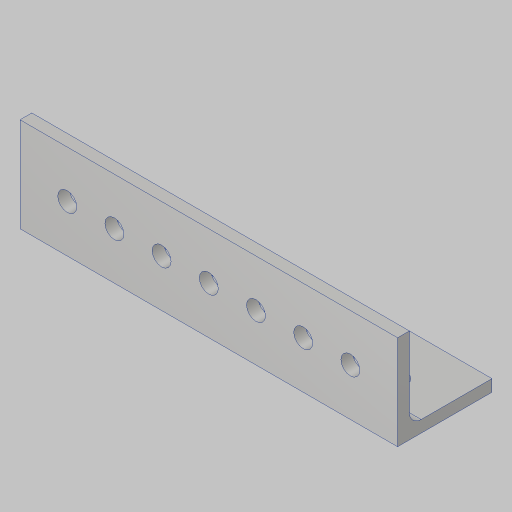
# Autodesk Inventor part: GI - 008
Saved by Autodesk Inventor 2023.5 (Build 275446000, 446)
## iProperties
Created: 2025-01-26
Part Number: GI - 008
Material: Aluminum 6061
Document SubType Name: Modeling
Designer: slick
Density: 2.7 g/cm^3
Appearance: Aluminum - Flat
Author: slick
Autodesk Inventor part; units mm, degrees
ref_plane "YZ Plane" through (0, 0, 0) normal (1, 0, 0) x (0, 1, 0)
ref_plane "XZ Plane" through (0, 0, 0) normal (0, 1, 0) x (-1, 0, 0)
ref_plane "XY Plane" through (0, 0, 0) normal (0, 0, 1) x (1, 0, 0)
sketch "Sketch1" plane through (0, 0, 0) normal (1, 0, 0) x (0, 1, 0)
  line L0 (25.4, 0) -> (0, 0)
  line L1 (0, 0) -> (0, -25.4)
  line L2 (0, -25.4) -> (3.175, -25.4)
  line L3 (3.175, -25.4) -> (3.175, -3.175)
  line L4 (3.175, -3.175) -> (25.4, -3.175)
  line L5 (25.4, -3.175) -> (25.4, 0)
  dimension "d0" = 25.4
  dimension "d1" = 25.4
  dimension "d2" = 3.175
  constraints: 12 end point, 5 perpendicular, 1 horizontal, 1 vertical
  measures "d0" distance of L0.start L0.end
  measures "d1" distance of L0.end L1.end
  measures "d2" distance between parallel lines of L4 L0
extrude "Extrusion1" add sketch "Sketch1" along normal mid plane 101.6
fillet "Fillet1" radius 3.175 1 edges at (0, 3.175, -3.175)
sketch "Sketch2" plane through (-50.8, 0, 0) normal (0, 0, 1) x (1, 0, 0)
  line L0 (0, 0) -> (0, 25.4) projected
  line L1 (101.6, 0) -> (0, 0) projected
  point P0 (50.8, 0)
  point P1 (12.7, 12.7)
  point P2 (0, 12.7)
  point P3 (25.4, 12.7)
  point P4 (38.1, 12.7)
  point P5 (50.8, 12.7)
  point P6 (63.5, 12.7)
  point P7 (76.2, 12.7)
  point P8 (88.9, 12.7)
  dimension "d6" = 12.7
  dimension "d9" = 12.7
  constraints: 1 horizontal, 1 horizontal alignment, 1 midpoint, 6 other
  measures "d6" distance from line of L0 point (12.7, 12.7)
  measures "d9" distance of point (12.7, 12.7) point (25.4, 12.7)
hole "Hole1" at (-38.1, 12.7, 0) at (-25.4, 12.7, 0) at (-12.7, 12.7, 0) at (0, 12.7, 0) at (12.7, 12.7, 0) at (25.4, 12.7, 0) at (38.1, 12.7, 0) direction (0, 0, -1) diameter 5.1054 end through all clearance for "Flat Head Machine Screw (82)" size "#10" standard "Ansi Unified Screw Threads"
sketch "Sketch3" plane through (-50.8, 0, -25.4) normal (0, -1, 0) x (1, 0, 0)
  line L0 (0, 0) -> (0, 25.4) projected
  line L1 (101.6, 25.4) -> (0, 25.4) projected
  point P0 (50.8, 25.4)
  point P1 (12.7, 12.7)
  point P2 (0, 12.7)
  point P3 (25.4, 12.7)
  point P4 (38.1, 12.7)
  point P5 (50.8, 12.7)
  point P6 (63.5, 12.7)
  point P7 (76.2, 12.7)
  point P8 (88.9, 12.7)
  dimension "d21" = 12.7
  dimension "d24" = 12.7
  constraints: 1 horizontal, 1 horizontal alignment, 1 midpoint, 6 other
  measures "d21" distance from line of point (12.7, 12.7) L0
  measures "d24" distance of point (12.7, 12.7) point (25.4, 12.7)
hole "Hole2" at (-38.1, 0, -12.7) at (-25.4, 0, -12.7) at (-12.7, 0, -12.7) at (0, 0, -12.7) at (12.7, 0, -12.7) at (25.4, 0, -12.7) at (38.1, 0, -12.7) direction (0, 1, 0) diameter 5.1054 end through all clearance for "Flat Head Machine Screw (82)" size "#10" standard "Ansi Unified Screw Threads"
equation "\"d1\" = d0"
body "Solid1"
